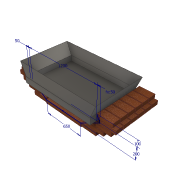
# Autodesk Inventor part: geo_pl
Saved by Autodesk Inventor 2019.1 (Build 231200000, 200)
## iProperties
Created: 2019-11-25
Part Number: geo_pl
Material: Concrete
Document SubType Name: Modeling
Designer: jjespitia
Density: 2.40731 g/cm^3
Appearance: Framing Steel
Author: jjespitia
Autodesk Inventor part; units mm, degrees
ref_plane "YZ Plane" through (0, 0, 0) normal (1, 0, 0) x (0, 1, 0)
ref_plane "XZ Plane" through (0, 0, 0) normal (0, 1, 0) x (-1, 0, 0)
ref_plane "XY Plane" through (0, 0, 0) normal (0, 0, 1) x (1, 0, 0)
sketch "Sketch1" plane through (0, 0, 0) normal (0, 0, 1) x (1, 0, 0)
  line L0 (-600, 0) -> (-650, -100)
  line L1 (-650, -100) -> (-325, -300)
  line L2 (-325, -300) -> (325, -300)
  line L3 (325, -300) -> (650, -100)
  line L4 (650, -100) -> (600, 0)
  line L5 (-600, 0) -> (-600, -100)
  line L6 (-600, -100) -> (600, -100)
  line L7 (600, -100) -> (600, 0)
  point P0 (0, 0)
  point P1 (0, -100)
  point P2 (0, -300)
  dimension "d0" = 650
  dimension "d1" = 200
  dimension "d2" = 1200
  dimension "d3" = 50
  dimension "d4" = 50
  dimension "d5" = 100
  constraints: 16 end point, 3 horizontal alignment, 2 midpoint, 2 perpendicular, 2 vertical alignment, 1 horizontal, 1 parallel, 1 vertical
  measures "d0" distance of L1.end L2.end
  measures "d1" distance between parallel lines of L2 L6
  measures "d2" distance of L5.end L6.end
  measures "d3" distance from line of L0.end L5
  measures "d4" distance from line of L7 L3.end
  measures "d5" distance of L6.end L4.end
sketch "Sketch2" plane through (0, 0, 0) normal (0, 0, 1) x (1, 0, 0)
  line L0 (-600, 0) -> (-650, -100) construction
  line L1 (-600, 0) -> (-600, -100) construction
  line L2 (-650, -100) -> (-325, -300) construction
  line L3 (-325, -300) -> (325, -300) construction
  line L4 (325, -300) -> (650, -100) construction
  line L5 (600, -100) -> (600, 0) construction
  line L6 (650, -100) -> (600, 0) construction
  line L7 (-600, -100) -> (600, -100) construction
  line L8 (-890, -70) -> (-650, -70)
  line L9 (-650, -70) -> (-650, -130)
  line L10 (-650, -130) -> (-890, -130)
  line L11 (-890, -130) -> (-890, -70)
  line L12 (2756.009, 105.6783) -> (3138.5717, 105.6783)
  line L13 (3138.5717, 105.6783) -> (3138.5717, -54.5407)
  line L14 (3138.5717, -54.5407) -> (2756.009, -54.5407)
  line L15 (2756.009, -54.5407) -> (2756.009, 105.6783)
  line L16 (-840, 0) -> (-600, 0)
  line L17 (-600, 0) -> (-600, -60)
  line L18 (-600, -60) -> (-840, -60)
  line L19 (-840, -60) -> (-840, 0)
  line L20 (-825, -140) -> (-585, -140)
  line L21 (-585, -140) -> (-585, -200)
  line L22 (-585, -200) -> (-825, -200)
  line L23 (-825, -200) -> (-825, -140)
  line L24 (-711.25, -210) -> (-471.25, -210)
  line L25 (-471.25, -210) -> (-471.25, -270)
  line L26 (-471.25, -270) -> (-711.25, -270)
  line L27 (-711.25, -270) -> (-711.25, -210)
  line L28 (-591.7811, -283.5193) -> (-351.7811, -283.5193)
  line L29 (-351.7811, -283.5193) -> (-351.7811, -343.5193)
  line L30 (-351.7811, -343.5193) -> (-591.7811, -343.5193)
  line L31 (-591.7811, -343.5193) -> (-591.7811, -283.5193)
  line L32 (-341.7811, -300) -> (341.7811, -300)
  line L33 (341.7811, -300) -> (341.7811, -360)
  line L34 (341.7811, -360) -> (-341.7811, -360)
  line L35 (-341.7811, -360) -> (-341.7811, -300)
  line L36 (0, -100) -> (0, -50)
  line L37 (600, 0) -> (600, -100) construction
  line L38 (890, -70) -> (650, -70)
  line L39 (650, -70) -> (650, -130)
  line L40 (650, -130) -> (890, -130)
  line L41 (890, -130) -> (890, -70)
  line L42 (600, 0) -> (600, -60)
  line L43 (600, -60) -> (840, -60)
  line L44 (840, 0) -> (600, 0)
  line L45 (840, -60) -> (840, 0)
  line L46 (585, -140) -> (585, -200)
  line L47 (585, -200) -> (825, -200)
  line L48 (825, -140) -> (585, -140)
  line L49 (825, -200) -> (825, -140)
  line L50 (471.25, -210) -> (471.25, -270)
  line L51 (471.25, -270) -> (711.25, -270)
  line L52 (711.25, -210) -> (471.25, -210)
  line L53 (711.25, -270) -> (711.25, -210)
  line L54 (351.7811, -283.5193) -> (351.7811, -343.5193)
  line L55 (351.7811, -343.5193) -> (591.7811, -343.5193)
  line L56 (591.7811, -283.5193) -> (351.7811, -283.5193)
  line L57 (591.7811, -343.5193) -> (591.7811, -283.5193)
  point P0 (0, 0)
  point P1 (-471.25, -87.3103)
  point P2 (-351.7811, -36.4756)
  point P3 (650, -100)
  point P4 (471.25, -87.3103)
  point P5 (351.7811, -36.4756)
  dimension "d6" = 60
  dimension "d7" = 240
  dimension "d8" = 60
  dimension "d9" = 240
  dimension "d10" = 60
  dimension "d11" = 240
  dimension "d12" = 10
  dimension "d13" = 10
  dimension "d14" = 60
  dimension "d15" = 240
  dimension "d16" = 10
  dimension "d17" = 60
  dimension "d18" = 240
  dimension "d19" = 13.5193
  dimension "d20" = 10
  dimension "d21" = 10
  constraints: 102 end point, 26 symmetric about line, 15 parallel, 7 horizontal, 7 perpendicular, 7 point on line, 3 midpoint, 1 collinear, 1 vertical
  measures "d6" distance between parallel lines of L8 L10
  measures "d7" distance of L8.start L8.end
  measures "d8" distance between parallel lines of L16 L18
  measures "d9" distance of L0.start L16.start
  measures "d10" distance between parallel lines of L20 L22
  measures "d11" distance of L20.start L21.start
  measures "d12" distance between parallel lines of L18 L8
  measures "d13" distance between parallel lines of L10 L20
  measures "d14" distance between parallel lines of L24 L26
  measures "d15" distance of L24.start L25.start
  measures "d16" distance between parallel lines of L22 L24
  measures "d17" distance between parallel lines of L28 L30
  measures "d18" distance of L28.start L29.start
  measures "d19" distance between parallel lines of L26 L28
  measures "d20" distance between parallel lines of L29 L35
  measures "d21" distance between parallel lines of L54 L33
extrude "Extrusion1" add sketch "Sketch2" against normal blind 120 contours L8 L9 L10 L11 | L16 L17 L18 L19 | L20 L21 L22 L23 | L24 L25 L26 L27 | L28 L29 L30 L31 | L32 L33 L34 L35 | L41 L40 L39 L38 | L44 L45 L43 L42 | L48 L49 L47 L46 | L52 L53 L51 L50 | L56 L57 L55 L54
pattern_linear "Rectangular Pattern1" count 6 spacing 130 along (0, 0, -1) of "Extrusion1"
sketch "Sketch3" plane through (0, 0, 0) normal (0, 0, 1) x (1, 0, 0)
  line L0 (-600, 0) -> (-600, -100) projected
  line L1 (-600, -100) -> (600, -100) projected
  line L2 (600, -100) -> (600, 0) projected
  line L3 (593.65, 0) -> (593.65, -93.65)
  line L4 (593.65, -93.65) -> (-593.65, -93.65)
  line L5 (-593.65, -93.65) -> (-593.65, 0)
  line L6 (-593.65, 0) -> (-674.4552, 200)
  line L7 (-595.4835, 0) -> (-676.2888, 200)
  line L8 (-595.4835, 0) -> (-600, 0)
  line L9 (600, 0) -> (595.4835, 0)
  line L10 (595.4835, 0) -> (676.2888, 200)
  line L11 (593.65, 0) -> (674.4552, 200)
  line L12 (-674.4552, 200) -> (-676.2888, 200)
  line L13 (676.2888, 200) -> (674.4552, 200)
  line L14 (-674.4552, 200) -> (674.4552, 200) construction
  point P0 (0, 200)
  point P1 (0, -100)
  dimension "d27" = 6.35
  dimension "d28" = 1.7
  dimension "d29" = 1.7
  dimension "d30" = 68
  dimension "d31" = 200
  constraints: 24 end point, 5 horizontal, 2 midpoint, 2 parallel, 1 horizontal alignment, 1 point on line, 1 vertical alignment, 2 other
  measures "d27" distance between parallel lines of L1 L4
  measures "d28" distance between parallel lines of L6 L7
  measures "d29" distance between parallel lines of L11 L10
  measures "d30" angle of L7 L8
  measures "d31" distance between parallel lines of L8 L12
extrude "Extrusion2" add sketch "Sketch3" against normal blind 700 and the other way blind 100 separate body
sketch "Sketch4" plane through (0, 0, 100) normal (0, 0, 1) x (1, 0, 0)
  line L0 (-600, 0) -> (-600, -100) projected
  line L1 (-600, -100) -> (600, -100) projected
  line L2 (600, -100) -> (600, 0) projected
  line L3 (600, 0) -> (595.4835, 0) projected
  line L4 (595.4835, 0) -> (676.2888, 200) projected
  line L5 (676.2888, 200) -> (674.4552, 200) construction
  line L6 (674.4552, 200) -> (593.65, 0) construction
  line L7 (593.65, 0) -> (593.65, -93.65) projected
  line L8 (593.65, -93.65) -> (-593.65, -93.65) projected
  line L9 (-593.65, -93.65) -> (-593.65, 0) projected
  line L10 (-593.65, 0) -> (-674.4552, 200) construction
  line L11 (-674.4552, 200) -> (-676.2888, 200) construction
  line L12 (-676.2888, 200) -> (-595.4835, 0) projected
  line L13 (-595.4835, 0) -> (-600, 0) projected
  line L14 (-676.2888, 200) -> (676.2888, 200)
  point P0 (0, 0)
  constraints: 3 point on line, 2 end point, 1 horizontal
extrude "Extrusion3" add sketch "Sketch4" along normal blind 1.7 bodies 2
sketch "Sketch5" plane through (0, 0, -700) normal (0, 0, -1) x (-1, 0, 0)
  line L0 (711.25, -210) -> (471.25, -210) projected
  line L1 (600, 0) -> (600, -100) projected
  line L2 (600, -100) -> (-600, -100) projected
  line L3 (-600, -100) -> (-600, 0) projected
  line L4 (-600, 0) -> (-595.4835, 0) projected
  line L5 (-595.4835, 0) -> (-676.2888, 200) projected
  line L6 (-676.2888, 200) -> (676.2888, 200) projected
  line L7 (676.2888, 200) -> (595.4835, 0) projected
  line L8 (595.4835, 0) -> (600, 0) projected
  point P0 (0, 0)
extrude "Extrusion4" add sketch "Sketch5" along normal blind 1.7 bodies 2
sketch "Sketch6" plane through (0, 0, 101.7) normal (0, 0, 1) x (1, 0, 0)
  line L0 (-600, 0) -> (600, 0)
  line L1 (600, 0) -> (600, -100)
  line L2 (600, -100) -> (-600, -100)
  line L3 (-600, -100) -> (-600, 0)
  point P0 (0, 0)
  constraints: 8 end point, 2 coincident, 2 parallel, 1 horizontal, 1 perpendicular
extrude "Extrusion5" add sketch "Sketch6" along normal blind 4.65 bodies 2
sketch "Sketch7" plane through (0, 0, -701.7) normal (0, 0, -1) x (-1, 0, 0)
  line L0 (-600, 0) -> (600, 0) projected
  line L1 (600, 0) -> (600, -100) projected
  line L2 (600, -100) -> (-600, -100) projected
  line L3 (-600, -100) -> (-600, 0) projected
  point P0 (0, 0)
extrude "Extrusion6" add sketch "Sketch7" along normal blind 4.65 bodies 2
extrude "Extrusion7" add sketch "Sketch1" along normal mid plane 1 separate body
equation "\"d4\" = d3"
equation "\"BendRadius\" = Thickness"
equation "\"BendReliefWidth\" = Thickness"
equation "\"BendReliefDepth\" = 0.5 * Thickness"
equation "\"CornerReliefSize\" = 4 * Thickness"
equation "\"MinimumRemnant\" = 2 * Thickness"
equation "\"TransitionRadius\" = BendRadius"
equation "\"JacobiRadiusSize\" = Thickness"
equation "\"GapSize\" = Thickness"
equation "\"Thickness\" = 0.5"
